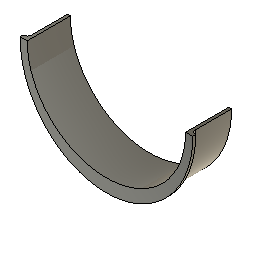
design (Autodesk Fusion 360 design; units mm, degrees)
Autodesk Fusion 360 part; units mm, degrees
sketch "Sketch1" plane through (0, 0, 0) normal (0, 0, 1) x (1, 0, 0) in component "滑块"
  line L0 (-45, 35) -> (45, 35)
  line L1 (45, 35) -> (45, -35)
  line L2 (45, -35) -> (-45, -35)
  line L3 (-45, -35) -> (-45, 35)
  line L4 (-45, 35) -> (45, -35) construction
  line L5 (-45, 20) -> (45, 20) construction
  line L6 (-50, 0) -> (50, 0) construction
  line L7 (-45, 17) -> (45, 17)
  line L8 (-45, 23) -> (45, 23)
  line L9 (-45, -17) -> (45, -17)
  line L10 (-45, -23) -> (45, -23)
  circle A0 centre (-20, 20) radius 1.6
  line L11 (0, 45) -> (0, -40) construction
  circle A1 centre (20, 20) radius 1.6
  circle A2 centre (20, -20) radius 1.6
  circle A3 centre (-20, -20) radius 1.6
  line L12 (20, 20) -> (-20, -20) construction
  line L13 (-20, 20) -> (20, -20) construction
  line L14 (-22.1213, 17.8787) -> (17.8787, -22.1213)
  line L15 (-17.8787, 22.1213) -> (22.1213, -17.8787)
  line L16 (17.8787, 22.1213) -> (-22.1213, -17.8787)
  line L17 (22.1213, 17.8787) -> (-17.8787, -22.1213)
  line L18 (20, 20) -> (45, 0) construction
  line L19 (20, -20) -> (45, 0) construction
  line L20 (-20, 20) -> (-45, 0) construction
  line L21 (-20, -20) -> (-45, 0) construction
  line L22 (-21.8741, 22.3426) -> (-49.8023, 0)
  line L23 (-21.8741, -22.3426) -> (-49.8023, 0)
  line L24 (-18.1259, -17.6574) -> (-43.1259, 2.3426)
  line L25 (-18.1259, 17.6574) -> (-43.1259, -2.3426)
  line L26 (18.1259, 17.6574) -> (43.1259, -2.3426)
  line L27 (21.8741, 22.3426) -> (46.8741, 2.3426)
  line L28 (21.8741, -22.3426) -> (46.8741, -2.3426)
  line L29 (18.1259, -17.6574) -> (43.1259, 2.3426)
  line L30 (25, 23) -> (25, -23)
  line L31 (-25, 23) -> (-25, -23)
  dimension "d1" = 90
  dimension "d2" = 70
  dimension "d20" = 20
  dimension "d21" = 3
  dimension "d22" = -3
  dimension "d23" = 3.2
  dimension "d24" = 20
  dimension "d27" = 3
  dimension "d28" = -3
  dimension "d29" = 3
  dimension "d30" = -3
  dimension "d33" = 3
  dimension "d34" = 3
  dimension "d35" = -3
  dimension "d36" = 3
  dimension "d37" = -3
  dimension "d38" = 3
  dimension "d39" = -3
  dimension "d40" = 5
  constraint horizontal L0
  constraint vertical L1
  constraint horizontal L2
  constraint vertical L3
  constraint midpoint origin L4
  constraint coincident L3 L5.start
  constraint coincident L1 L5.end
  constraint perpendicular L1 L5
  constraint perpendicular L3 L6
  constraint coincident L3 L9.start
  constraint coincident L1 L9.end
  constraint perpendicular L1 L9
  constraint coincident L3 L10.start
  constraint coincident L1 L10.end
  constraint perpendicular L1 L10
  constraint symmetric L6 L7 L9
  constraint symmetric L6 L8 L10
  constraint coincident L5 A0.centre
  constraint perpendicular L0 L11
  constraint coincident L5 A1.centre
  constraint symmetric L6 A0 A3
  constraint symmetric A0 L11 A1
  constraint symmetric L6 A1 A2
  constraint coincident A1.centre L12.start
  constraint coincident A3.centre L12.end
  constraint coincident A0.centre L13.start
  constraint coincident A2.centre L13.end
  constraint midpoint L1 L18.end
  constraint midpoint L3 L20.end
  constraint coincident L8 L30.start
  constraint coincident L10 L30.end
  constraint perpendicular L10 L30
  constraint coincident L8 L31.start
  constraint coincident L10 L31.end
  constraint perpendicular L10 L31
  constraint symmetric L11 L30 L31
  measures "d1" distance of L0.start L0.end
  measures "d2" distance of L0.start L2.end
  measures "d20" distance of L5 L6
  measures "d23" diameter of A0
  measures "d24" distance of A0.centre L11
  measures "d40" distance of A2.centre L30
extrude "Extrude5" add sketch "Sketch1" along normal blind 4 contours L3 L7 L8 L22 L31 | L1 L7 L8 L27 L30 | L7 L8 L30 L31 | L3 L7 L9 L22 L23 L24 L25 L31 | L7 L22 L31 | L1 L7 L9 L26 L27 L28 L29 L30 | L7 L27 L30 | L7 L14 L25 L31 | L7 L17 L26 L30 | L3 L9 L10 L23 L31 | L9 L23 L31 | L7 L14 L25 | L1 L9 L10 L28 L30 | L9 L28 L30 | L7 L17 L26 | L9 L16 L24 L31 | L9 L10 L30 L31 | L7 L14 L15 L16 L25 | L9 L15 L29 L30 | L7 L15 L16 L17 L26 | L9 L16 L24 | L14 L15 L16 L17 | L9 L14 L16 L17 L24 | L9 L15 L29 | L9 L14 L15 L17 L29 makes body 1 in component "滑块"
ref_plane "WorkPlane1" through (-45, 0, -0.5) normal (-1, 0, 0) x (0, 1, 0) in component "滑块"
sketch "Sketch2" plane through (-45, 0, -0.5) normal (-1, 0, 0) x (0, 1, 0) in component "滑块"
  circle A0 centre (0, -35.5) radius 27.5
  line L0 (-35, -0.5) -> (35, -0.5)
  line L1 (0, -60) -> (0, 10) construction
  circle A1 centre (0, -35.5) radius 30
  line L2 (30, -35.5) -> (30, -62)
  line L3 (-30, -35.5) -> (-30, -60)
  line L4 (33, -45.5) -> (-33, -45.5)
  line L5 (33, -45.5) -> (35, -0.5)
  line L6 (-33, -45.5) -> (-35, -0.5)
  point P0 (0, -45.5)
  dimension "d6" = 55
  dimension "d7" = 35
  dimension "d8" = 2.5
  dimension "d9" = 66
  dimension "d10" = 10
  constraint vertical L1
  constraint coincident A0.centre L1
  constraint coincident A1 L2.start
  constraint vertical L2
  constraint coincident A1 L3.start
  constraint vertical L3
  constraint tangent A1 L2
  constraint tangent A1 L3
  constraint horizontal L4
  constraint midpoint L4 P0
  constraint coincident L1 P0
  constraint coincident L0.end L5.end
  constraint coincident L0.start L6.end
  measures "d6" diameter of A0
  measures "d7" distance of A0.centre L0
  measures "d9" distance of L4.start L4.end
  measures "d10" distance of A0.centre L4
sketch "Sketch1 (2)" plane through (0, 0, 0) normal (0, 0, 1) x (1, 0, 0) in component "导轨"
  line L0 (-30, 50) -> (30, 50)
  line L1 (30, 50) -> (30, -50)
  line L2 (30, -50) -> (-30, -50)
  line L3 (-30, -50) -> (-30, 50)
  line L4 (-30, 50) -> (30, -50) construction
  line L5 (0, 75) -> (0, -65) construction
  line L6 (-30, 44) -> (30, 44) construction
  line L7 (-30, 5.5) -> (30, 5.5) construction
  circle A0 centre (19.325, 44) radius 3.5
  line L8 (17.75, 44) -> (20.9, 44) construction
  circle A1 centre (-19.325, 44) radius 3.5
  circle A2 centre (19.325, 5.5) radius 3.5
  circle A3 centre (-19.325, 5.5) radius 3.5
  line L9 (19.325, 44) -> (19.325, 5.5) construction
  line L10 (-30, -45) -> (30, -45)
  line L11 (-20.9, 50) -> (-20.9, -26.5)
  line L12 (-17.75, 50) -> (-17.75, -26.5)
  line L13 (17.75, 50) -> (17.75, -26.5)
  line L14 (20.9, 50) -> (20.9, -26.5)
  line L15 (-20.9, 12) -> (20.9, 12)
  line L16 (-20.9, -26.5) -> (20.9, -26.5)
  line L17 (-10.25, 44) -> (10.25, 44)
  line L18 (10.25, 44) -> (10.25, 12)
  line L19 (10.25, 12) -> (-10.25, 12)
  line L20 (-10.25, 12) -> (-10.25, 44)
  line L21 (-10.25, 5.5) -> (10.25, 5.5)
  line L22 (10.25, 5.5) -> (10.25, -26.5)
  line L23 (10.25, -26.5) -> (-10.25, -26.5)
  line L24 (-10.25, -26.5) -> (-10.25, 5.5)
  dimension "d53" = 60
  dimension "d54" = 100
  dimension "d55" = 35.5
  dimension "d56" = 41.8
  dimension "d57" = 6
  dimension "d58" = 38.5
  dimension "d59" = 7
  dimension "d73" = 5
  dimension "d82" = 32
  dimension "d83" = 32
  dimension "d86" = 20.5
  dimension "d87" = 20.5
  constraint horizontal L0
  constraint vertical L1
  constraint horizontal L2
  constraint vertical L3
  constraint midpoint origin L4
  constraint vertical L5
  constraint coincident L0 L13.start
  constraint perpendicular L2 L13
  constraint coincident L0 L14.start
  constraint perpendicular L2 L14
  constraint coincident L0 L12.start
  constraint perpendicular L2 L12
  constraint coincident L0 L11.start
  constraint perpendicular L2 L11
  constraint symmetric L5 L12 L13
  constraint symmetric L5 L11 L14
  constraint coincident L3 L6.start
  constraint coincident L1 L6.end
  constraint perpendicular L1 L6
  constraint coincident L3 L7.start
  constraint coincident L1 L7.end
  constraint perpendicular L1 L7
  constraint coincident L6 A0.centre
  constraint coincident L6 L8.start
  constraint coincident L8.start L13
  constraint coincident L6 L8.end
  constraint coincident L8.end L14
  constraint midpoint A0.centre L8
  constraint coincident L6 A1.centre
  constraint coincident L7 A2.centre
  constraint coincident L7 A3.centre
  constraint equal A0 A2
  constraint coincident A0.centre L9.start
  constraint perpendicular L7 L9
  constraint coincident A2.centre L9.end
  constraint symmetric L5 A0 A1
  constraint symmetric L5 A2 A3
  constraint coincident L3 L10.start
  constraint coincident L1 L10.end
  constraint perpendicular L1 L10
  constraint coincident L11 L15.start
  constraint coincident L14 L15.end
  constraint perpendicular L14 L15
  constraint perpendicular L14 L16
  constraint coincident L12.end L16
  constraint coincident L13.end L16
  constraint horizontal L17
  constraint vertical L18
  constraint horizontal L19
  constraint vertical L20
  constraint coincident L15 L18.end
  constraint coincident L6 L17.start
  constraint horizontal L21
  constraint vertical L22
  constraint horizontal L23
  constraint vertical L24
  constraint coincident L16 L22.end
  constraint coincident L7 L21.start
  constraint symmetric L5 L18 L20
  constraint symmetric L5 L22 L24
  measures "d53" distance of L0.start L0.end
  measures "d54" distance of L0.start L2.end
  measures "d55" distance of L12 L13
  measures "d56" distance of L11 L14
  measures "d57" distance of L0 L6
  measures "d58" distance of L6 L7
  measures "d59" diameter of A0
  measures "d73" distance of L2 L10
  measures "d82" distance of L6 L15
  measures "d83" distance of L7 L16
  measures "d86" distance of L18 L20
  measures "d87" distance of L22 L24
extrude "Extrude3" add sketch "Sketch1 (2)" along normal blind 15 separate body contours L1 L2 L3 L10 makes body 2 in component "导轨"
extrude "Extrude2" add sketch "Sketch1 (2)" along normal blind 5 contours L0 L1 L3 A0 A1 A2 A3 L10 L11 L14 L16 L23 | L0 A1 L11 L12 | L1 L2 L3 L10 | L0 A0 A1 L12 L13 L15 L17 L18 L20 | L0 A0 L13 L14 | A3 L11 L12 L15 | A2 A3 L12 L13 L15 L16 L19 L21 L22 L24 | A2 L13 L14 L15 bodies 2 in component "导轨"
ref_plane "WorkPlane2" through (0, -15, 7.5) normal (0, -1, 0) x (1, 0, 0) in component "导轨"
fillet "Fillet1" radius 2 1 edges at (0, -45, 5) on bodies 2 in component "导轨"
sketch "Sketch3" plane through (0, -50, 0) normal (0, -1, 0) x (1, 0, 0) in component "导轨"
  line L0 (30, 0) -> (30, 15)
  line L1 (30, 15) -> (-30, 15)
  line L2 (-30, 15) -> (-30, 0)
  line L3 (-30, 0) -> (30, 0)
  line L4 (-30, 12) -> (30, 12)
  dimension "d77" = 3
  constraint coincident L2 L4.start
  constraint coincident L0 L4.end
  constraint perpendicular L0 L4
  measures "d77" distance of L1 L4
extrude "Extrude4" add sketch "Sketch3" against normal blind 7 contours L0 L1 L2 L4 bodies 2 in component "导轨"
chamfer "Chamfer4" distance 2 angle 45 1 edges at (0, -45, 12) on bodies 2 in component "导轨"
fillet "Fillet2" radius 6 1 edges at (0, -50, 15) on bodies 2 in component "导轨"
chamfer "Chamfer5" distance 1.9 angle 50 8 edges at (-20.9, 26.4372, 5) (-17.75, 26.4372, 5) (17.75, 26.4372, 5) (20.9, 26.4372, 5) (17.75, -12.0628, 5) (20.9, -12.0628, 5) (-17.75, -12.0628, 5) (-20.9, -12.0628, 5) measured on face at (-3.4167, -37.5, 5) measured on face at (-3.4167, -37.5, 5) measured on face at (-3.4167, -37.5, 5) measured on face at (-3.4167, -37.5, 5) measured on face at (-3.4167, -37.5, 5) measured on face at (-3.4167, -37.5, 5) measured on face at (-3.4167, -37.5, 5) measured on face at (-3.4167, -37.5, 5) on bodies 2 in component "导轨"
fillet "Fillet3" radius 5 8 edges at (-10.25, 44, 2.5) (-10.25, 5.5, 2.5) (10.25, 5.5, 2.5) (10.25, 12, 2.5) (-10.25, 12, 2.5) (10.25, 44, 2.5) (10.25, -26.5, 2.5) (-10.25, -26.5, 2.5) on bodies 2 in component "导轨"
fillet "Fillet4" radius 1.5 8 edges at (-20.9, 12, 1.3678) (-20.9, -26.5, 1.3678) (17.75, 12, 1.3678) (17.75, -26.5, 1.3678) (-17.75, -26.5, 1.3678) (-17.75, 12, 1.3678) (20.9, 12, 1.3678) (20.9, -26.5, 1.3678) on bodies 2 in component "导轨"
sketch "Sketch1 (3)" plane through (0, 0, 0) normal (0, 1, 0) x (1, 0, 0) in component "垫环"
  circle A0 centre (0, 0) radius 27.5
  line L0 (0, -50) -> (0, 50) construction
  ellipse E0 centre (0, 0) end of major axis (0, 30.5) minor radius 28.5
  line L1 (0, -30.5) -> (0, 30.5)
  line L2 (28.5, 0) -> (-28.5, 0)
  line L3 (-29.994, 0) -> (29.996, 0)
  spline S0 degree 3 poles (0, -32) (5.5838, -32) (11.1567, -30.294) (15.8836, -27.1477) (20.7177, -23.9299) (24.651, -19.2184) (27.0905, -13.7485) (29.5621, -8.2068) (30.4934, -1.9046) (29.7437, 4.1743) (28.9991, 10.2123) (26.5983, 16.0112) (22.902, 20.6709) (19.3022, 25.2089) (14.4841, 28.6519) (9.1586, 30.4726) (3.877, 32.2784) (-1.885, 32.4803) (-7.2677, 31.047) (-12.7294, 29.5926) (-17.7799, 26.4611) (-21.6616, 22.14) (-25.7016, 17.6427) (-28.4615, 11.8722) (-29.5099, 5.7611) (-30.5444, -0.2693) (-29.9109, -6.6115) (-27.7049, -12.2766) (-25.4546, -18.0553) (-21.5723, -23.1085) (-16.6795, -26.5991) (-12.0764, -29.8829) (-6.5958, -31.7736) (-1.0484, -31.9805) (-0.6991, -31.9935) (-0.3495, -32) (0, -32) knots -3.141593 -3.141593 -3.141593 -3.141593 -2.585167 -2.585167 -2.585167 -2.016107 -2.016107 -2.016107 -1.439577 -1.439577 -1.439577 -0.866931 -0.866931 -0.866931 -0.309233 -0.309233 -0.309233 0.243873 0.243873 0.243873 0.805104 0.805104 0.805104 1.389226 1.389226 1.389226 1.965642 1.965642 1.965642 2.553617 2.553617 2.553617 3.106761 3.106761 3.106761 3.141593 3.141593 3.141593 3.141593
  dimension "d90" = 55
  dimension "d91" = 61
  dimension "d92" = 57
  dimension "d93" = 1.5
  constraint coincident A0.centre E0.centre
  constraint vertical L0
  constraint parallel L0 L1
  constraint coincident E0 L1.start
  constraint coincident E0 L1.end
  constraint coincident E0 L2.start
  constraint coincident E0 L2.end
  constraint parallel L2 L3
  constraint coincident S0 L3.start
  constraint coincident L2.end L3
  constraint coincident S0 L3.end
  constraint coincident L2.start L3
  measures "d90" diameter of A0
  measures "d91" distance of E0
extrude "Extrude1" add sketch "Sketch1 (3)" along normal blind 15 separate body contours A0 E0 L1 L2 L3 | A0 E0 L1 L2 L3 picked at (2.2159, 28.3598) picked at (-6.403, 27.6724) makes body 3 in component "垫环"
extrude "Extrude2'" add sketch "Sketch1 (3)" along normal blind 1 contours E0 L3 S0 picked at (23.5493, 18.0155) bodies 3 in component "垫环"
fillet "Fillet1'" radius 1.5 1 edges at (0, 1, -30.5) on bodies 3 in component "垫环"
extrude "Extrude1'" [suppressed] in component "导轨"
ref_plane "WorkPlane1" through (0, 40, 0) normal (0, 1, 0) x (1, 0, 0) in component "导轨"
sketch "Sketch2 (2)" plane through (0, 40, 0) normal (0, 1, 0) x (1, 0, 0) in component "导轨"
  line L0 (-30, -5) -> (30, -5)
  line L1 (30, 0) -> (-30, 0)
  line L2 (30, 0) -> (30, -5)
  line L3 (-30, 0) -> (-30, -5)
  line L4 (-20.9, 0) -> (-20.9, -5)
  line L5 (-17.75, 0) -> (-17.75, -5)
  line L6 (17.75, 0) -> (17.75, -5)
  line L7 (20.9, 0) -> (20.9, -5)
  point P0 (-20.9, 0)
  point P1 (-17.75, 0)
  point P2 (17.75, 0)
  point P3 (20.9, 0)
  constraint coincident P0 L4.start
  constraint coincident L0 L4.end
  constraint perpendicular L0 L4
  constraint coincident P1 L5.start
  constraint coincident L0 L5.end
  constraint perpendicular L0 L5
  constraint coincident P2 L6.start
  constraint coincident L0 L6.end
  constraint perpendicular L0 L6
  constraint coincident P3 L7.start
  constraint coincident L0 L7.end
  constraint perpendicular L0 L7
extrude "Extrude2''" [suppressed] in component "滑块"
ref_plane "WorkPlane2" through (45, 0, -0.5) normal (1, 0, 0) x (0, -1, 0) in component "滑块"
sketch "Sketch3 (2)" plane through (45, 0, -0.5) normal (1, 0, 0) x (0, 1, 0) in component "滑块"
  circle A0 centre (0, 35.5) radius 19
  circle A1 centre (0, 35.5) radius 20.5
  circle A2 centre (0, 35.5) radius 24
  line L0 (35, 0.5) -> (-35, 0.5)
  line L1 (35, 0.5) -> (-35, 0.5)
  line L2 (-35, 0.5) -> (-35, -0.5)
  line L3 (-35, -0.5) -> (35, -0.5)
  line L4 (35, -0.5) -> (35, 0.5)
  line L5 (-35, 0.5) -> (-23.0708, 42.1136)
  line L6 (35, 0.5) -> (23.0708, 42.1136)
  point P0 (0, 35.5)
  dimension "d14" = 38
  dimension "d15" = 1.5
  dimension "d16" = 5
  constraint coincident P0 A0.centre
  constraint coincident L0.end L1.end
  constraint coincident A2 L5.end
  constraint tangent A2 L5
  constraint coincident L0.start L1.start
  constraint coincident A2 L6.end
  constraint tangent A2 L6
  measures "d14" diameter of A0
extrude "Extrude3'" [suppressed] in component "滑块"
chamfer "Chamfer1" [suppressed] in component "滑块"
chamfer "Chamfer2" [suppressed] in component "滑块"
fillet "Fillet1''" [suppressed] in component "滑块"
ref_plane "WorkPlane3" through (1, -23, 2) normal (0, -1, 0) x (1, 0, 0) in component "滑块"
sketch "Sketch5" plane through (1, -23, 2) normal (0, -1, 0) x (1, 0, 0) in component "滑块"
  line L0 (36, -2) -> (36, 2)
  line L1 (36, 2) -> (-36, 2)
  line L2 (-36, 2) -> (-36, -2)
  line L3 (-36, -2) -> (36, -2)
  line L4 (44, -2) -> (44, 37.7349)
  line L5 (44, 37.7349) -> (36, 37.7349)
  line L6 (36, 37.7349) -> (36, -2)
  line L7 (36, -2) -> (44, -2)
  line L8 (-46, 40.5) -> (-46, -2)
  line L9 (-46, -2) -> (-36, -2)
  line L10 (-36, -2) -> (-36, 40.5)
  line L11 (-36, 40.5) -> (-46, 40.5)
  line L12 (25, -2) -> (36, 17.0526)
  line L13 (25, -2) -> (45.5699, -2) construction
  point P0 (19, -2)
  point P1 (-21, -2)
  dimension "d44" = 60
  dimension "d45" = 6
  constraint horizontal L13
  constraint coincident L3 L12.start
  constraint coincident L6 L12.end
  measures "d44" angle of L12 L13
  measures "d45" distance of P0 L12.start
extrude "Extrude6" [suppressed] in component "滑块"
sketch "Sketch4" plane through (0, -23, 0) normal (0, -1, 0) x (1, 0, 0) in component "滑块"
  line L0 (37, 0) -> (37, 4)
  line L1 (37, 4) -> (-35, 4)
  line L2 (-35, 4) -> (-35, 0)
  line L3 (-35, 0) -> (37, 0)
  line L4 (25, 0) -> (45, 34.641)
  line L5 (25, 0) -> (62.1196, 0) construction
  line L6 (45, 0) -> (45, 44)
  line L7 (45, 0) -> (-45, 0) construction
  point P0 (20, 0)
  point P1 (45, 0)
  dimension "d41" = 60
  dimension "d42" = 5
  constraint horizontal L5
  constraint coincident L3 L4.start
  constraint coincident L5 P1
  constraint perpendicular L5 L6
  constraint coincident L6 P1
  constraint coincident L4.end L6
  constraint perpendicular L2 L7
  measures "d41" angle of L4 L5
  measures "d42" distance of L4.start P0
extrude "Extrude4'" [suppressed] in component "滑块"
component "滑块" placed x (1, 0, 0) y (0, 1, 0) z (0, 0, 1) at (0, 0, 0)
component "导轨" placed x (1, 0, 0) y (0, 1, 0) z (0, 0, 1) at (0, 0, 0)
component "垫环" placed x (1, 0, 0) y (0, 1, 0) z (0, 0, 1) at (0, 0, 0)
equation "d83 = ( d82 )"
equation "d86 = ( d55 - 15 mm )"
equation "d87 = ( d86 )"
